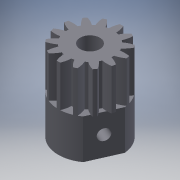
# Autodesk Inventor part: Spur Gear1
Saved by Autodesk Inventor 2016 (Build 200138000, 138)
## iProperties
Created: 2016-12-04
Part Number: Spur Gear1
Material: Steel
Document SubType Name: Modeling
Designer: William
Categories: <?xml version="1.0" encoding="UTF-16"?> <MemberInstance><Categories><FamilyTemplate><FamilyTemplateParameter ValueType="xs:double" Id="1" ObjectReferenceKey="da_z" ObjectType="kUserParameterObject"/><FamilyTemplateParameter ValueType="xs:double" Id="2" ObjectReferenceKey="da_b" ObjectType="kUserParameterObject"/><FamilyTemplateParameter ValueType="xs:double" Id="3" ObjectReferenceKey="da_beta" ObjectType="kUserParameterObject"/><FamilyTemplateParameter ValueType="xs:double" Id="4" ObjectReferenceKey="da_da" ObjectType="kUserParameterObject"/><FamilyTemplateParameter ValueType="xs:double" Id="5" ObjectReferenceKey="da_aw" ObjectType="kUserParameterObject"/><FamilyTemplateParameter ValueType="xs:string" Id="6" ObjectReferenceKey="EAIAABAAAACIAQAAAAAAAIAAAAAAAAAA" ObjectType="83910656" SubObjectId="SurfaceGeometry"/></FamilyTemplate><ParamToTemplateMap><ParamToTemplate CategoryParameter="//CategoryParameter[@InternalName='046C89C9-8512-4d59-83FE-43B91F4F132A']" TemplateParameter="1"/><ParamToTemplate CategoryParameter="//CategoryParameter[@InternalName='2552DF32-E462-4b46-AEBF-C6C7768E72AC']" TemplateParameter="2"/><ParamToTemplate CategoryParameter="//CategoryParameter[@InternalName='C9EE641D-15FC-4fae-A226-E94C4372FDD7']" TemplateParameter="3"/><ParamToTemplate><ParamToTemplate CategoryParameter="//CategoryParameter[@InternalName='00B6519A-459B-49c7-AD84-2E56D39A5744']" ConstantValue="0.000000"/></ParamToTemplate><ParamToTemplate><ParamToTemplate CategoryParameter="//CategoryParameter[@InternalName='04B31F0E-C7A6-4894-AA32-9629BEFACF47']" ConstantValue="1.000000"/></ParamToTemplate><ParamToTemplate><ParamToTemplate CategoryParameter="//CategoryParameter[@InternalName='43CBEC2E-7847-49e7-A936-2F7889FCB2D9']" ConstantValue="0.250000"/></ParamToTemplate><ParamToTemplate><ParamToTemplate CategoryParameter="//CategoryParameter[@InternalName='B1EFC894-105D-4ebd-86BF-FA20ED196853']" ConstantValue="0.350000"/></ParamToTemplate><ParamToTemplate><ParamToTemplate CategoryParameter="//CategoryParameter[@InternalName='51175063-3D10-4879-93E8-6246FE8B403D']" ConstantValue="2060000000.000000"/></ParamToTemplate><ParamToTemplate><ParamToTemplate CategoryParameter="//CategoryParameter[@InternalName='A3A52E27-4454-46a9-B0BD-C932399B70AF']" ConstantValue="0.300000"/></ParamToTemplate><ParamToTemplate><ParamToTemplate CategoryParameter="//CategoryParameter[@InternalName='91B76062-C214-41d9-B1B9-14D2AB99603D']" ConstantValue="0.150000"/></ParamToTemplate><ParamToTemplate><ParamToTemplate CategoryParameter="//CategoryParameter[@InternalName='374E806E-8B8A-4dda-A9AA-1039D6500AD2']" ConstantValue="6.666667"/></ParamToTemplate><ParamToTemplate><ParamToTemplate CategoryParameter="//CategoryParameter[@InternalName='2D373A89-B862-43d6-8D0B-0CBF12AB9F6C']" ConstantValue="0.349066"/></ParamToTemplate><ParamToTemplate CategoryParameter="//CategoryParameter[@InternalName='37777632-D6A2-4fac-9D53-DB8ACD95C989']" TemplateParameter="4"/><ParamToTemplate CategoryParameter="//CategoryParameter[@InternalName='FD1017F1-B727-4f7e-9707-0F86F1FF9423']" TemplateParameter="5"/><ParamToTemplate><ParamToTemplate CategoryParameter="//CategoryParameter[@InternalName='9E1B4470-B2D3-4ff1-B813-535BB4CDF51A']" ConstantValue="3520000.000000"/></ParamToTemplate><ParamToTemplate><ParamToTemplate CategoryParameter="//CategoryParameter[@InternalName='F8452263-BFF6-458c-9FB1-07C4B99E95CD']" ConstantValue="11400000.000000"/></ParamToTemplate><ParamToTemplate><ParamToTemplate CategoryParameter="//CategoryParameter[@InternalName='3E3BB259-FD49-497f-8171-6EBC954A3479']" ConstantValue="2.000000"/></ParamToTemplate><ParamToTemplate CategoryParameter="//CategoryParameter[@InternalName='27C3BAF2-7550-4e4b-AE2C-0DB134B7D9B7']" TemplateParameter="6"/></ParamToTemplateMap><Category DisplayName="Gear" InternalName="DC85795E-93AB-48d5-8EEE-5A27447B64BD" Mnemonic="Gear"><CategoryParameter DisplayName="z" InternalName="046C89C9-8512-4d59-83FE-43B91F4F132A" Mnemonic="z"/><CategoryParameter DisplayName="b" InternalName="2552DF32-E462-4b46-AEBF-C6C7768E72AC" Mnemonic="b"/><CategoryParameter DisplayName="||b|" InternalName="C9EE641D-15FC-4fae-A226-E94C4372FDD7" Mnemonic="beta"/><CategoryParameter DisplayName="x" InternalName="00B6519A-459B-49c7-AD84-2E56D39A5744" Mnemonic="x"/><CategoryParameter DisplayName="a*" InternalName="04B31F0E-C7A6-4894-AA32-9629BEFACF47" Mnemonic="a"/><CategoryParameter DisplayName="c*" InternalName="43CBEC2E-7847-49e7-A936-2F7889FCB2D9" Mnemonic="c"/><CategoryParameter DisplayName="r|.f|*" InternalName="B1EFC894-105D-4ebd-86BF-FA20ED196853" Mnemonic="rf"/><CategoryParameter DisplayName="E" InternalName="51175063-3D10-4879-93E8-6246FE8B403D" Mnemonic="E"/><CategoryParameter DisplayName="||m|" InternalName="A3A52E27-4454-46a9-B0BD-C932399B70AF" Mnemonic="mi"/><Category DisplayName="SpurGear" InternalName="26C5A22E-A91E-4dfd-A3B3-23CCAFAE1764" Mnemonic="SpurGear"><CategoryParameter DisplayName="m" InternalName="91B76062-C214-41d9-B1B9-14D2AB99603D" Mnemonic="m"/><CategoryParameter DisplayName="P" InternalName="374E806E-8B8A-4dda-A9AA-1039D6500AD2" Mnemonic="PP"/><CategoryParameter DisplayName="||a|" InternalName="2D373A89-B862-43d6-8D0B-0CBF12AB9F6C" Mnemonic="alpha"/><CategoryParameter DisplayName="d|.a|" InternalName="37777632-D6A2-4fac-9D53-DB8ACD95C989" Mnemonic="da"/><CategoryParameter DisplayName="a|.w|" InternalName="FD1017F1-B727-4f7e-9707-0F86F1FF9423" Mnemonic="aw"/><CategoryParameter DisplayName="||s||.Flim|" InternalName="9E1B4470-B2D3-4ff1-B813-535BB4CDF51A" Mnemonic="sFlim"/><CategoryParameter DisplayName="||s||.Hlim|" InternalName="F8452263-BFF6-458c-9FB1-07C4B99E95CD" Mnemonic="sHlim"/><CategoryParameter DisplayName="type" InternalName="3E3BB259-FD49-497f-8171-6EBC954A3479" Mnemonic="type"/><CategoryParameter DisplayName="PitchDiameter" InternalName="27C3BAF2-7550-4e4b-AE2C-0DB134B7D9B7" Mnemonic="IDS_PITCHDIAM"/></Category></Category></Categories></MemberInstance>
Density: 1 g/cm^3
Appearance: Steel
CustomPartVersion: 1
Author: William
Autodesk Inventor part; units mm, degrees
sketch "Sketch1" plane through (0, 0, 0) normal (0, 0, 1) x (1, 0, 0)
  circle A0 centre (0, 0) radius 8.25
  dimension "d0" = 16.5
  constraints: 1 centre point
  measures "d0" diameter of A0
extrude "Extrusion1" add sketch "Sketch1" along normal blind 10.4
ref_plane "Work Plane2" through (0, 0, 5.2) normal (0, 0, 1) x (1, 0, 0)
sketch "Sketch2" plane through (0, 0, 0) normal (0, 0, -1) x (-1, 0, 0)
  circle A0 centre (0, 0) radius 8.25 projected
  circle A1 centre (0, 0) radius 6.75
  dimension "d3" = 13.5
  constraints: 1 centre point, 1 coincident
  measures "d3" diameter of A1
surface extrude "Pitch Diameter" sketch "Sketch2" against normal through all shown no curves A1
ref_plane "Work Plane8" through (0, 0, 0) normal (0.9396926, 0.3420201, 0) x (0, 0, 1)
ref_plane "Work Plane9" through (0, 0, 0) normal (1, 0, 0) x (0, 1, 0)
spur gear teeth "Spur Gear" teeth 9 pitch diameter 13.5 tip diameter 16.5 root diameter 9.75 face width 10.4 start plane through (0, 0, 0) normal (0, 0, -1) x (-1, 0, 0)
sketch "Sketch5" plane through (0, 0, 0) normal (0, 0, -1) x (-1, 0, 0)
  line L0 (5.4643, 7.4635) -> (9.2409, 0.4111)
  line L1 (-9.2409, -0.4111) -> (-5.4643, -7.4635)
  arc A0 (-5.4643, -7.4635) -> (9.2409, 0.4111) centre (0, 0) ccw
  arc A1 (5.4643, 7.4635) -> (-9.2409, -0.4111) centre (0, 0) ccw
  dimension "d63" = 9.25
  dimension "d64" = 9.25
  dimension "d65" = 8
  dimension "d66" = 8
  constraints: 4 end point, 4 point on circle, 2 centre point, 1 coincident, 1 parallel
  measures "d63" radius of A1
  measures "d64" radius of A0
  measures "d65" distance of L0.start L0.end
  measures "d66" distance of L1.start L1.end
extrude "Extrusion4" add sketch "Sketch5" along normal blind 10
sketch "Sketch6" plane through (0, 0, -10) normal (0, 0, -1) x (-0.8815592, 0.4720735, 0)
  circle A0 centre (0, 0) radius 2.5
  dimension "d58" = 5
  constraints: 1 centre point, 1 coincident
  measures "d58" diameter of A0
extrude "Extrusion5" cut sketch "Sketch6" against normal up to next
sketch "Sketch7" plane through (5.4643, -7.4635, 0) normal (0.8815592, -0.4720735, 0) x (0, 0, -1)
  circle A0 centre (4, 4) radius 1.4
  line L0 (0, 7.5564) -> (0, 8) projected
  line L1 (0, 0) -> (0, 8) projected
  line L2 (0, 8) -> (10, 8) projected
  point P0 (0, 4)
  point P1 (0, 4.5274)
  point P2 (0, 6.0736)
  point P3 (0, 6.8423)
  dimension "d67" = 2.8
  dimension "d73" = 4
  dimension "d74" = 4
  constraints: 1 centre point
  measures "d67" diameter of A0
  measures "d73" distance from line of L1 A0.centre
  measures "d74" distance from line of L2 A0.centre
extrude "Extrusion6" cut sketch "Sketch7" against normal up to surface (16.6808 mm away)
sketch "Sketch8" plane through (0, 0, 10.4) normal (0, 0, 1) x (1, 0, 0)
  circle A0 centre (0, 0) radius 2.5 projected
  arc A1 (5.8336, 5.8336) -> (4.732, 6.758) centre (0, 0) ccw projected
  arc A2 (-6.758, -4.732) -> (-3.4471, -3.4471) centre (-7.7909, 2.8379) ccw projected
  arc A3 (-3.4471, -3.4471) -> (-2.7962, -3.9934) centre (0, 0) ccw projected
  arc A4 (-2.7962, -3.9934) -> (-3.4866, -7.477) centre (4.1477, -7.1798) ccw projected
  arc A5 (-3.4866, -7.477) -> (-2.1353, -7.9689) centre (0, 0) ccw projected
  arc A6 (-2.1353, -7.9689) -> (-0.4249, -4.8564) centre (-7.7924, -2.834) ccw projected
  arc A7 (-0.4249, -4.8564) -> (0.4249, -4.8564) centre (0, 0) ccw projected
  arc A8 (0.4249, -4.8564) -> (2.1353, -7.9689) centre (7.7924, -2.834) ccw projected
  arc A9 (2.1353, -7.9689) -> (3.4866, -7.477) centre (0, 0) ccw projected
  arc A10 (3.4866, -7.477) -> (2.7962, -3.9934) centre (-4.1477, -7.1798) ccw projected
  arc A11 (2.7962, -3.9934) -> (3.4471, -3.4471) centre (0, 0) ccw projected
  arc A12 (3.4471, -3.4471) -> (6.758, -4.732) centre (7.7909, 2.8379) ccw projected
  arc A13 (6.758, -4.732) -> (7.477, -3.4866) centre (0, 0) ccw projected
  arc A14 (7.477, -3.4866) -> (4.7089, -1.2617) centre (1.4378, -8.1661) ccw projected
  arc A15 (4.7089, -1.2617) -> (4.8564, -0.4249) centre (0, 0) ccw projected
  arc A16 (4.8564, -0.4249) -> (8.2186, 0.719) centre (4.1441, 7.1819) ccw projected
  arc A17 (8.2186, 0.719) -> (7.9689, 2.1353) centre (0, 0) ccw projected
  arc A18 (7.9689, 2.1353) -> (4.4183, 2.0603) centre (6.3505, -5.3314) ccw projected
  arc A19 (4.4183, 2.0603) -> (3.9934, 2.7962) centre (0, 0) ccw projected
  arc A20 (3.9934, 2.7962) -> (5.8336, 5.8336) centre (-1.4419, 8.1654) ccw projected
  arc A21 (4.732, 6.758) -> (2.0603, 4.4183) centre (8.2917, -0.0021) ccw projected
  arc A22 (2.0603, 4.4183) -> (1.2617, 4.7089) centre (0, 0) ccw projected
  arc A23 (1.2617, 4.7089) -> (0.719, 8.2186) centre (-6.3532, 5.3282) ccw projected
  arc A24 (-0.719, 8.2186) -> (-1.2617, 4.7089) centre (6.3532, 5.3282) ccw projected
  arc A25 (-1.2617, 4.7089) -> (-2.0603, 4.4183) centre (0, 0) ccw projected
  arc A26 (-2.0603, 4.4183) -> (-4.732, 6.758) centre (-8.2917, -0.0021) ccw projected
  arc A27 (-5.8336, 5.8336) -> (-3.9934, 2.7962) centre (1.4419, 8.1654) ccw projected
  arc A28 (-3.9934, 2.7962) -> (-4.4183, 2.0603) centre (0, 0) ccw projected
  arc A29 (-4.4183, 2.0603) -> (-7.9689, 2.1353) centre (-6.3505, -5.3314) ccw projected
  arc A30 (-7.9689, 2.1353) -> (-8.2186, 0.719) centre (0, 0) ccw projected
  arc A31 (-8.2186, 0.719) -> (-4.8564, -0.4249) centre (-4.1441, 7.1819) ccw projected
  arc A32 (-4.8564, -0.4249) -> (-4.7089, -1.2617) centre (0, 0) ccw projected
  arc A33 (-4.7089, -1.2617) -> (-7.477, -3.4866) centre (-1.4378, -8.1661) ccw projected
  arc A34 (-7.477, -3.4866) -> (-6.758, -4.732) centre (0, 0) ccw projected
  arc A35 (-4.732, 6.758) -> (-5.8336, 5.8336) centre (0, 0) ccw projected
  arc A36 (0.719, 8.2186) -> (-0.719, 8.2186) centre (0, 0) ccw projected
extrude "Extrusion7" add sketch "Sketch8" along normal blind 2.5
equation "\"d0\" = da_da"
equation "\"d1\" = da_b"
equation "\"d3\" = da_dw"
equation "\"d16\" = da_aw"
equation "\"d66\" = d65"
equation "\"d43\" = da_aw"
equation "\"d46\" = da_aw"
equation "\"da_da\" = 16.5"
equation "\"da_b\" = 10.4"
equation "\"da_dw\" = 13.5"
equation "\"da_aw\" = 75"
body "Solid1"
body "Srf1"
